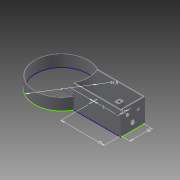
# Autodesk Inventor part: Pump enclosure MM0312
Saved by Autodesk Inventor 2013 SP2 (Build 170200200, 200)
## iProperties
Created: 2015-07-01
Part Number: Pump enclosure MM0312
Material: Generic
Document SubType Name: Modeling
Designer: kthorn
Density: 1 g/cm^3
Author: kthorn
Autodesk Inventor part; units mm, degrees
ref_plane "YZ Plane" through (0, 0, 0) normal (1, 0, 0) x (0, 1, 0)
ref_plane "XZ Plane" through (0, 0, 0) normal (0, 1, 0) x (-1, 0, 0)
ref_plane "XY Plane" through (0, 0, 0) normal (0, 0, 1) x (1, 0, 0)
sketch "Sketch1" plane through (0, 0, 0) normal (0, 0, 1) x (1, 0, 0)
  circle A0 centre (0, 0) radius 45.75
  circle A1 centre (0, 0) radius 46.75
  line L0 (45.75, -0.0157) -> (46.75, -0.0157) construction
  line L1 (42.7149, 19) -> (121.75, 19)
  line L2 (121.75, 19) -> (121.75, -19)
  line L3 (121.75, -19) -> (42.7149, -19)
  line L4 (41.768, 21) -> (123.75, 21)
  line L5 (123.75, 21) -> (123.75, -21)
  line L6 (123.75, -21) -> (41.768, -21)
  line L7 (82.759, 21) -> (82.759, 19) construction
  line L8 (121.75, 0) -> (123.75, 0) construction
  line L9 (98.0367, -19) -> (98.0367, -21) construction
  line L10 (0, 0) -> (121.75, 0) construction
  line L11 (41.768, 21) -> (40.6456, 21)
  line L12 (41.768, -21) -> (40.6456, -21)
  dimension "d0" = 91.5
  dimension "d2" = 1
  dimension "d3" = 75
  dimension "d4" = 38
  dimension "d5" = 2
  constraints: 26 end point, 8 point on circle, 5 perpendicular, 4 parallel, 3 horizontal, 3 midpoint, 3 point on line, 2 centre point, 2 equal length, 1 coincident
  measures "d0" diameter of A0
  measures "d2" distance of L0.end L0.start
  measures "d3" distance from line of L2 L0.end
  measures "d4" distance of L1.end L2.end
  measures "d5" distance of L7.start L7.end
extrude "Extrusion1" add sketch "Sketch1" along normal blind 20 contours A0 L11 A1 L12 | A0 L12 A1 L11
extrude "Extrusion2" add sketch "Sketch1" along normal blind 2 contours L4 L5 L6 A1 L3 L2 L1 | L1 L2 L3 A1
extrude "Extrusion9" add sketch "Sketch1" along normal blind 40 contours A0 L11 A1 L12 | L4 L5 L6 A1 L3 L2 L1 picked at (42.2726, -18.1004)
sketch "Sketch8" plane through (123.75, -21, 0) normal (1, 0, 0) x (0, 0, -1)
  line L0 (0, 0) -> (0, 42) projected
  line L1 (0, 42) -> (-40, 42) projected
  line L2 (-40, 0) -> (-40, 42) projected
  line L3 (0, 0) -> (-40, 0) projected
  circle A0 centre (-12, 21) radius 4.05
  line L4 (-12, 21) -> (-12, 42) construction
  line L5 (-12, 21) -> (-12, 0) construction
  circle A1 centre (-28, 30) radius 3.25
  circle A2 centre (-28, 12) radius 3.25
  line L6 (-28, 30) -> (-28, 12) construction
  line L7 (-40, 21) -> (-28, 21) construction
  point P0 (0, 21)
  dimension "d40" = 8.1
  dimension "d42" = 12
  dimension "d43" = 6.5
  dimension "d44" = 12
  dimension "d61" = 18
  constraints: 8 end point, 3 centre point, 2 midpoint, 2 perpendicular, 2 point on line, 1 collinear, 1 equal radius, 1 horizontal, 1 parallel
  measures "d40" diameter of A0
  measures "d42" distance from line of L0 L4.start
  measures "d43" diameter of A1
  measures "d44" distance of L7.start L7.end
  measures "d61" distance of L6.start L6.end
extrude "Extrusion10" cut sketch "Sketch8" against normal up to surface (2 mm away) contours A0 | A1 | A2
sketch "Sketch9" plane through (0, 0, 2) normal (0, 0, 1) x (1, 0, 0)
  arc A0 (42.7149, -19) -> (42.7149, 19) centre (0, 0) ccw projected
  line L0 (42.7149, -19) -> (121.75, -19) projected
  line L1 (46.75, 0) -> (81.75, 0) construction
  line L2 (81.75, 19) -> (89.75, 19)
  line L3 (89.75, 19) -> (89.75, 9.25)
  line L4 (89.75, 9.25) -> (81.75, 9.25)
  line L5 (81.75, 9.25) -> (81.75, 19)
  line L6 (81.75, -19) -> (89.75, -19)
  line L7 (89.75, -19) -> (89.75, -9.25)
  line L8 (89.75, -9.25) -> (81.75, -9.25)
  line L9 (81.75, -9.25) -> (81.75, -19)
  line L10 (81.75, 19) -> (81.75, -19) construction
  line L11 (42.7149, 19) -> (121.75, 19) projected
  line L12 (89.75, -19) -> (81.75, -19)
  dimension "d49" = 35
  dimension "d52" = 18.5
  dimension "d53" = 8
  constraints: 22 end point, 4 parallel, 4 point on line, 3 perpendicular, 2 equal length, 2 horizontal, 1 collinear, 1 midpoint, 1 point on circle
  measures "d49" distance of L1.start L1.end
  measures "d52" distance of L7.end L3.end
  measures "d53" distance of L3.end L4.end
extrude "Extrusion11" add sketch "Sketch9" along normal blind 15
sketch "Sketch10" plane through (0, 0, 17) normal (0, 0, 1) x (1, 0, 0)
  line L0 (81.75, 19) -> (89.75, 19) projected
  line L1 (81.75, 19) -> (81.75, 9.25) projected
  line L2 (81.75, 9.25) -> (89.75, 9.25) projected
  line L3 (89.75, 9.25) -> (89.75, 19) projected
  line L4 (89.75, -19) -> (89.75, -9.25) projected
  line L5 (89.75, -9.25) -> (81.75, -9.25) projected
  line L6 (81.75, -9.25) -> (81.75, -19) projected
  line L7 (89.75, -19) -> (81.75, -19) projected
  circle A0 centre (85.75, -14.125) radius 2.1
  circle A1 centre (85.75, 14.125) radius 2.1
  line L8 (89.75, 19) -> (81.75, 9.25) construction
  line L9 (89.75, -9.25) -> (81.75, -19) construction
  point P0 (0, 0)
  dimension "d58" = 4.2
  constraints: 4 end point, 2 centre point, 2 midpoint, 1 equal radius, 1 parallel
  measures "d58" diameter of A1
extrude "Extrusion12" cut sketch "Sketch10" against normal blind 5 contours A0 | A1
body "Solid1"
